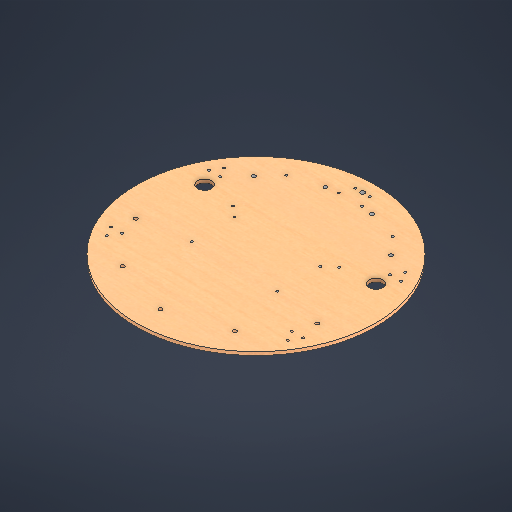
# Autodesk Inventor part: layer6_new
Saved by Autodesk Inventor 2026 (Build 300175050, 175E)
## iProperties
Created: 2025-06-05
Part Number: layer6_new
Material: Generic
Document SubType Name: Modeling
Designer: satom
Density: 1 g/cm^3
Appearance: Default
Author: satom
Autodesk Inventor part; units mm, degrees
ref_plane "YZ Plane" through (0, 0, 0) normal (1, 0, 0) x (0, 1, 0)
ref_plane "XZ Plane" through (0, 0, 0) normal (0, 1, 0) x (-1, 0, 0)
ref_plane "XY Plane" through (0, 0, 0) normal (0, 0, 1) x (1, 0, 0)
sketch "Sketch1" plane through (0, 0, 0) normal (0, 1, 0) x (-1, 0, 0)
  circle A0 centre (0, 0) radius 177
  dimension "d0" = 354
  constraints: 1 centre point, 1 coincident
  measures "d0" diameter of A0
extrude "Extrusion1" add sketch "Sketch1" along normal blind 5
sketch "Sketch2" plane through (0, 5, 0) normal (0, 1, 0) x (1, 0, 0)
  line L0 (0, 0) -> (153.2865, -88.5) construction
  circle A0 centre (0, 0) radius 177 construction
  line L1 (-177, 0) -> (177, 0) construction
  circle A1 centre (142.288, -82.15) radius 1.7
  line L2 (142.288, -82.15) -> (134.0391, -77.3875) construction
  circle A2 centre (142.288, -72.625) radius 1.7
  circle A3 centre (134.0391, -67.8625) radius 1.7
  circle A4 centre (125.7902, -72.625) radius 1.7
  circle A5 centre (125.7902, -82.15) radius 1.7
  circle A6 centre (134.0391, -86.9125) radius 1.7
  line L3 (0, 177) -> (0, -177) construction
  circle A7 centre (0, 0) radius 177 construction
  circle A8 centre (-142.288, -72.625) radius 1.7
  circle A9 centre (-125.7902, -72.625) radius 1.7
  circle A10 centre (-134.0391, -86.9125) radius 1.7
  circle A11 centre (0, 0) radius 177 construction
  circle A12 centre (142.288, 72.625) radius 1.7
  circle A13 centre (125.7902, 72.625) radius 1.7
  circle A14 centre (134.0391, 86.9125) radius 1.7
  circle A15 centre (-125.7902, 72.625) radius 1.7
  circle A16 centre (-142.288, 72.625) radius 1.7
  circle A17 centre (-134.0391, 86.9125) radius 1.7
  dimension "d3" = 30
  dimension "d4" = 3.4
  dimension "d5" = 12.7
  dimension "d6" = 9.525
  dimension "d9" = 360
  constraints: 17 centre point, 9 symmetric about line, 8 end point, 5 point on circle, 2 point on line, 1 horizontal, 1 perpendicular, 24 other
  measures "d3" angle of L1 L0
  measures "d4" diameter of A1
  measures "d5" distance of L0.end L2.start
  measures "d6" distance of L2.start L2.end
extrude "Standoffs" cut sketch "Sketch2" against normal through all contours A2 | A4 | A6 | A8 | A9 | A10 | A12 | A13 | A14 | A15 | A16 | A17
sketch "Sketch3" plane through (0, 5, 0) normal (0, 1, 0) x (1, 0, 0)
  circle A0 centre (-127, 50.8) radius 10.16
  circle A1 centre (127, 50.8) radius 10.16
  circle A2 centre (0, 0) radius 177 construction
  circle A3 centre (0, 0) radius 177 construction
  line L0 (0, 0) -> (0, 177) construction
  line L1 (0, 0) -> (177, 0) construction
  line L2 (0, 0) -> (-177, 0) construction
  dimension "d13" = 20.32
  dimension "d14" = 20.32
  dimension "d19" = 127
  dimension "d20" = 127
  dimension "d21" = 50.8
  dimension "d22" = 50.8
  constraints: 6 end point, 3 point on circle, 2 centre point, 1 horizontal, 1 point on line, 1 vertical
  measures "d13" diameter of A0
  measures "d14" diameter of A1
  measures "d19" distance from line of L0 A0.centre
  measures "d20" distance from line of L0 A1.centre
  measures "d21" distance from line of L2 A0.centre
  measures "d22" distance from line of L1 A1.centre
extrude "Wires" cut sketch "Sketch3" against normal through all
sketch "Sketch4" plane through (0, 5, 0) normal (0, 1, 0) x (1, 0, 0)
  circle A0 centre (0, -141.44) radius 2.667
  circle A1 centre (0, 0) radius 177 construction
  line L0 (0, 0) -> (0, -177) construction
  line L1 (0, -177) -> (48.7641, -177) construction
  circle A2 centre (83.1363, -114.4274) radius 2.667
  circle A3 centre (-83.1363, -114.4274) radius 2.667
  circle A4 centre (134.5174, -43.7074) radius 2.667
  circle A5 centre (-134.5174, -43.7074) radius 2.667
  circle A6 centre (-34.3789, 137.1983) radius 2.667
  circle A7 centre (-101.628, 98.3718) radius 2.667
  line L2 (0, 0) -> (-34.3789, 137.1983) construction
  line L3 (0, 177) -> (0, -177) construction
  line L4 (-101.628, 98.3718) -> (0, 0) construction
  circle A8 centre (34.3789, 137.1983) radius 2.667
  circle A9 centre (101.628, 98.3718) radius 2.667
  dimension "d25" = 5.334
  dimension "d28" = 35.56
  dimension "d31" = 144
  dimension "d67" = 5.334
  dimension "d68" = 5.334
  dimension "d69" = 14.067
  dimension "d70" = 141.44
  dimension "d71" = 45.933
  dimension "d73" = 141.44
  constraints: 10 end point, 9 centre point, 2 point on circle, 2 symmetric about line, 2 vertical, 1 horizontal, 1 point on line, 11 other
  measures "d25" diameter of A0
  measures "d28" distance from line of L1 A0.centre
  measures "d67" diameter of A6
  measures "d68" diameter of A7
  measures "d69" angle of L3 L2
  measures "d70" distance of L0.start L2.end
  measures "d71" angle of L3 L4
  measures "d73" distance of L4.start L0.start
extrude "Zip Ties" cut sketch "Sketch4" against normal through all
sketch "Sketch5" plane through (0, 5, 0) normal (0, 1, 0) x (1, 0, 0)
  circle A0 centre (-63.5, 31.75) radius 1.7
  circle A1 centre (0, 0) radius 177 construction
  line L0 (-177, 0) -> (177, 0) construction
  line L1 (0, -177) -> (0, 177) construction
  circle A2 centre (63.5, 31.75) radius 1.7
  circle A3 centre (-63.5, -31.75) radius 1.7
  circle A4 centre (63.5, -31.75) radius 1.7
  dimension "d35" = 3.4
  dimension "d36" = 63.5
  dimension "d37" = 31.75
  constraints: 4 centre point, 4 end point, 4 point on circle, 3 symmetric about line, 2 horizontal, 1 perpendicular, 1 vertical, 3 other
  measures "d35" diameter of A0
  measures "d36" distance from line of L1 A0.centre
  measures "d37" distance from line of L0 A0.centre
extrude "LiDAR" cut sketch "Sketch5" along normal through all both and the other way through all
sketch "Sketch6" plane through (0, 5, 0) normal (0, 1, 0) x (1, 0, 0)
  circle A0 centre (-17.145, 139.7) radius 1.7
  circle A1 centre (0, 0) radius 177 construction
  line L0 (-177, 0) -> (177, 0) construction
  line L1 (0, -196.4897) -> (0, 177) construction
  circle A2 centre (17.145, 139.7) radius 1.7
  dimension "d40" = 3.4
  dimension "d41" = 17.145
  dimension "d42" = 139.7
  constraints: 4 end point, 3 point on circle, 2 centre point, 2 horizontal, 1 perpendicular, 1 symmetric about line, 1 vertical, 1 other
  measures "d40" diameter of A0
  measures "d41" distance from line of L1 A0.centre
  measures "d42" distance from line of L0 A0.centre
extrude "Astra Camera" cut sketch "Sketch6" against normal through all
sketch "Sketch7" plane through (0, 5, 0) normal (0, 1, 0) x (1, 0, 0)
  circle A0 centre (0, 0) radius 177 construction
  line L0 (-177, 0) -> (177, 0) construction
  line L1 (0, 177) -> (0, -177) construction
  circle A1 centre (-78.745, 44.45) radius 1.7
  circle A2 centre (-78.745, 123.61) radius 1.7
  circle A3 centre (78.745, 44.45) radius 1.7
  circle A4 centre (78.745, 123.61) radius 1.7
  dimension "d45" = 3.4
  dimension "d46" = 44.45
  dimension "d47" = 78.745
  dimension "d48" = 3.4
  dimension "d50" = 78.745
  dimension "d51" = 79.16
  constraints: 4 centre point, 4 end point, 4 point on circle, 2 horizontal, 2 symmetric about line, 1 perpendicular, 1 vertical, 2 other
  measures "d45" diameter of A1
  measures "d46" distance from line of L0 A1.centre
  measures "d47" distance from line of L1 A1.centre
  measures "d48" diameter of A2
  measures "d50" distance from line of L1 A2.centre
  measures "d51" distance of A2.centre A1.centre
extrude "Display" cut sketch "Sketch7" against normal through all
sketch "Sketch8" plane through (0, 5, 0) normal (0, 1, 0) x (1, 0, 0)
  circle A0 centre (-10.795, 157.95) radius 1.7
  circle A1 centre (10.795, 157.95) radius 1.7
  circle A2 centre (0, 157.95) radius 3.175
  circle A3 centre (0, 0) radius 177 construction
  line L0 (0, 177) -> (46.0077, 177) construction
  line L1 (0, 177) -> (0, -177) construction
  dimension "d54" = 3.4
  dimension "d55" = 3.4
  dimension "d57" = 6.35
  dimension "d59" = 19.05
  dimension "d60" = 19.05
  dimension "d61" = 19.05
  dimension "d63" = 10.795
  dimension "d64" = 10.795
  constraints: 4 end point, 3 centre point, 2 point on circle, 1 horizontal, 1 point on line, 1 tangent, 1 vertical
  measures "d54" diameter of A0
  measures "d55" diameter of A1
  measures "d57" diameter of A2
  measures "d59" distance from line of L0 A1.centre
  measures "d60" distance from line of L0 A2.centre
  measures "d61" distance from line of L0 A0.centre
  measures "d63" distance of A2.centre A0.centre
  measures "d64" distance of A2.centre A1.centre
extrude "Arducam" cut sketch "Sketch8" against normal through all
equation "\"d0\" = robot_diameter"
equation "\"d1\" = hardboard_thickness"
equation "\"d4\" = m3_clearance"
equation "\"d14\" = d13"
equation "\"d22\" = d21"
equation "\"d67\" = d25"
equation "\"d68\" = d25"
equation "\"d73\" = d70"
equation "\"d35\" = m3_clearance"
equation "\"d40\" = m3_clearance"
equation "\"d45\" = m3_clearance"
equation "\"d48\" = d49"
equation "\"d50\" = d47"
equation "\"d54\" = m3_clearance"
equation "\"d55\" = d56"
equation "\"d60\" = d59"
equation "\"d61\" = d59"
equation "\"m3_heat_set_insert\" = 4"
equation "\"m3_clearance\" = 3.4"
equation "\"m3_heat_set_depth\" = 7"
equation "\"robot_diameter\" = 354"
equation "\"hardboard_thickness\" = 5"
equation "\"d49\" = 3.4"
equation "\"d56\" = 3.4"
body "Solid1"
